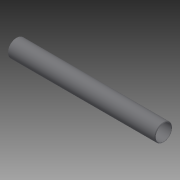
# Autodesk Inventor part: 09R-9.31350C
Saved by Autodesk Inventor 2014 (Build 180170000, 170)
## iProperties
Category: PARTsolutions
Company: BIMBA
Created: 2014-01-18
Part Number: 09R-9.31350C
Material: Generic
Catalog Web Link: www.cadenas.de
Description: Tube-Original Line - Standard Air Cylinders
Vendor: BIMBA
Document SubType Name: Standard Catalog Part
Designer: Andrew Toennies
Manufacturer: BIMBA
Density: 1 g/cm^3
Appearance: RGB(180.00000447034725,180.00000447034725,180.00000447034725)
PSOL_IDENT_0: {$CADENAS_DATA\23d-libs\bimba\bimba\bimba_imperial\bimba_full_line\original_line_cylinders\standard_
PSOL_IDENT_1: air_cylinders\tube.prj},192 {VTYP=3D},{NB=09R-9.31350C},{LINA=09R-9.31350C},{NN=Tube},{DATE=20.08.20
PSOL_IDENT_2: 11 07:16:50},{GEOMDATE=18.02.2011 00:00:00},{VERSION=},{LINEID=60},{LINESUBID=-1},{WBVAR=MNT,ACTING,
PSOL_IDENT_3: NR,L,FOURHOLES,SR}  {NB=09R-9.31350C},{LINA=09R-9.31350C},{KT=DUMMY},{PN=09R-9.31350C},{BORE=1.06250
PSOL_IDENT_4: 000},{BOREPN=09},{MNT=},{MNTALG='' , 'Front Nose' , 'BF' , 'Front Block' , 'BFT' , 'Front Trunnion'
PSOL_IDENT_5: , 'A' , 'Adjustable Stroke'},{ACTING=R},{ACTINGALG= '' , 'Single Acting' , 'R' , 'Reverse/Double Act
PSOL_IDENT_6: ing' },{NR=},{NRALG= '' , 'N/A' },{L=9.3135},{OD=1.1130},{ODN=1.1130},{ODP=1.1130},{ODB=1.1410},{ID=
PSOL_IDENT_7: 1.0715},{DV=0.00000000},{LV=0.00000000},{LV1=0.00000000},{G=0.0300},{FOURHOLES=0},{AA=0.3750},{BB=0.
PSOL_IDENT_8: 0940},{SR=C},{SRALG= 'C' , 'Carbon Steel Rod' , 'SR' , '303 Stainless Steel Rod' , '' , '303 Stainle
PSOL_IDENT_9: ss Steel Rod'}
CNS_NN: Tube
CNS_NT: Original Line - Standard Air Cylinders
CNS_NB: 09R-9.31350C
CNS_NBSYN: $PN.
CNS_LINA: 09R-9.31350C
CNS_PN: 09R-9.31350C
CNS_BORE: 1 1/16
CNS_BOREPN: 09
CNS_MNT: Front Nose
CNS_MNTALG: '' , 'Front Nose' , 'BF' , 'Front Block' , 'BFT' , 'Front Trunnion' , 'A' , 'Adjustable Stroke'
CNS_ACTING: Reverse/Double Acting
CNS_ACTINGALG: '' , 'Single Acting' , 'R' , 'Reverse/Double Acting'
CNS_NR: N/A
CNS_NRALG: '' , 'N/A'
CNS_L: 9.3135
CNS_OD: 1.1130
CNS_ODN: 1.1130
CNS_ODP: 1.1130
CNS_ODB: 1.1410
CNS_ID: 1.0715
CNS_DV: 0.00000000
CNS_LV: 0.00000000
CNS_LV1: 0.00000000
CNS_G: 0.0300
CNS_FOURHOLES: 0
CNS_AA: 0.3750
CNS_BB: 0.0940
CNS_SR: Carbon Steel Rod
CNS_SRALG: 'C' , 'Carbon Steel Rod' , 'SR' , '303 Stainless Steel Rod' , '' , '303 Stainless Steel Rod'
SUPPLIER: BIMBA
ARTICLENO: 09R-9.31350C
BOMINFO: 09R-9.31350C
CREATOR: CADENAS GmbH
Title: 09R-9.31350C
Author: Cadenas PARTsolutions
Comments: Original Line - Standard Air Cylinders
Autodesk Inventor part; units mm, degrees
sketch "Sketch_1" plane through (0, 0, 0) normal (0, 0, 1) x (1, 0, 0)
  line L0 (236.5629, 0) -> (0, 0)
  arc A0 (-0.6395, 13.2842) -> (-0.6395, 13.1046) centre (-0.5497, 13.1944) ccw
  line L1 (-0.6395, 13.1046) -> (-0.381, 12.846)
  line L2 (-0.381, 12.846) -> (0, 12.846)
  line L3 (0, 12.846) -> (0.762, 13.608)
  line L4 (0.762, 13.608) -> (235.8009, 13.608)
  line L5 (235.8009, 13.608) -> (236.5629, 12.846)
  line L6 (236.5629, 12.846) -> (236.9439, 12.846)
  line L7 (236.9439, 12.846) -> (237.2024, 13.1046)
  arc A1 (237.2024, 13.1046) -> (237.2024, 13.2842) centre (237.1126, 13.1944) ccw
  line L8 (237.2024, 13.2842) -> (236.5747, 13.9119)
  arc A2 (236.5747, 13.9119) -> (236.0358, 14.1351) centre (236.0359, 13.3731) ccw
  line L9 (236.0358, 14.1351) -> (0.5271, 14.1351)
  arc A3 (0.5271, 14.1351) -> (-0.0118, 13.9119) centre (0.527, 13.3731) ccw
  line L10 (-0.0118, 13.9119) -> (-0.6395, 13.2842)
  constraints: 22 end point, 8 point on circle, 4 centre point
revolve "Revolution1" add sketch "Sketch_1" angle 360 about axis through (236.5629, 0, 0) along (1, 0, 0)
ref_plane "cp1_XY" through (118.2814, 14.1351, 0) normal (1, 0, 0) x (0, 0, -1)
ref_plane "cp1_YZ" through (118.2814, 14.1351, 0) normal (0, 0, -1) x (0, 1, 0)
ref_plane "cp1_ZX" through (118.2814, 14.1351, 0) normal (0, 1, 0) x (1, 0, 0)
ref_plane "cp2_XY" through (118.2814, 0, -14.1351) normal (1, 0, 0) x (0, 0, -1)
ref_plane "cp2_YZ" through (118.2814, 0, -14.1351) normal (0, 0, -1) x (0, 1, 0)
ref_plane "cp2_ZX" through (118.2814, 0, -14.1351) normal (0, 1, 0) x (1, 0, 0)
ref_plane "cp3_XY" through (118.2814, -14.1351, 0) normal (1, 0, 0) x (0, 0, -1)
ref_plane "cp3_YZ" through (118.2814, -14.1351, 0) normal (0, 0, -1) x (0, 1, 0)
ref_plane "cp3_ZX" through (118.2814, -14.1351, 0) normal (0, 1, 0) x (1, 0, 0)
ref_plane "cp4_XY" through (118.2814, 0, 14.1351) normal (1, 0, 0) x (0, 0, -1)
ref_plane "cp4_YZ" through (118.2814, 0, 14.1351) normal (0, 0, -1) x (0, 1, 0)
ref_plane "cp4_ZX" through (118.2814, 0, 14.1351) normal (0, 1, 0) x (1, 0, 0)
ref_plane "tube_front_XY" through (0, 0, 0) normal (1, 0, 0) x (0, 0, -1)
ref_plane "tube_front_YZ" through (0, 0, 0) normal (0, 0, -1) x (0, 1, 0)
ref_plane "tube_front_ZX" through (0, 0, 0) normal (0, 1, 0) x (1, 0, 0)
ref_plane "tube_rear_XY" through (236.5629, 0, 0) normal (1, 0, 0) x (0, 0, -1)
ref_plane "tube_rear_YZ" through (236.5629, 0, 0) normal (0, 0, -1) x (0, 1, 0)
ref_plane "tube_rear_ZX" through (236.5629, 0, 0) normal (0, 1, 0) x (1, 0, 0)
body "Solid1"
